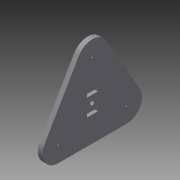
# Autodesk Inventor part: RibEnd
Saved by Autodesk Inventor 2015 (Build 190159000, 159)
## iProperties
Created: 2014-11-09
Part Number: RibEnd
Material: Generic
Document SubType Name: Modeling
Designer: Ryan
Density: 1 g/cm^3
Appearance: Default
Author: Ryan
Autodesk Inventor part; units mm, degrees
ref_plane "YZ Plane" through (0, 0, 0) normal (1, 0, 0) x (0, 1, 0)
ref_plane "XZ Plane" through (0, 0, 0) normal (0, 1, 0) x (-1, 0, 0)
ref_plane "XY Plane" through (0, 0, 0) normal (0, 0, 1) x (1, 0, 0)
sketch "Sketch1" plane through (0, 0, 0) normal (1, 0, 0) x (0, 1, 0)
  line L0 (2.9851, 0) -> (0, 0) construction
  line L1 (0, 0) -> (0, 4.2) construction
  circle A0 centre (0, 0) radius 1.425
  circle A1 centre (25.125, 0) radius 10
  circle A2 centre (-12.5625, 21.7589) radius 10
  circle A3 centre (-12.5625, -21.7589) radius 10
  line L2 (-7.5625, 30.4191) -> (30.125, 8.6603)
  line L3 (-22.5625, 21.7589) -> (-22.5625, -21.7589)
  line L4 (30.125, -8.6603) -> (-7.5625, -30.4191)
  line L5 (0, 0) -> (-12.5625, 21.7589) construction
  line L6 (-12.5625, 21.7589) -> (-12.5625, -21.7589) construction
  line L7 (-12.5625, 21.7589) -> (25.125, 0) construction
  line L8 (6.5, 3.5) -> (4.5, 3.5)
  line L9 (4.5, 3.5) -> (4.5, -3.5)
  line L10 (4.5, -3.5) -> (6.5, -3.5)
  line L11 (6.5, -3.5) -> (6.5, 3.5)
  line L12 (-4.5, 3.5) -> (-6.5, 3.5)
  line L13 (-6.5, 3.5) -> (-6.5, -3.5)
  line L14 (-6.5, -3.5) -> (-4.5, -3.5)
  line L15 (-4.5, -3.5) -> (-4.5, 3.5)
  dimension "d0" = 25.125
  dimension "d1" = 25.125
  dimension "d2" = 60
  dimension "d3" = 20
  dimension "d4" = 20
  dimension "d5" = 2.85
  dimension "d6" = 2
  dimension "d7" = 7
  dimension "d8" = 4.5
  constraints: 32 end point, 6 point on circle, 6 tangent, 4 centre point, 4 parallel, 3 horizontal, 2 perpendicular, 2 vertical, 1 coincident, 1 point on line, 1 symmetric about line, 6 other
  measures "d0" distance of L7.end L0.end
  measures "d1" distance of L5.start L5.end
  measures "d2" angle of L6 L7
  measures "d3" diameter of A1
  measures "d4" diameter of A3
  measures "d5" diameter of A0
  measures "d6" distance of L9.end L10.end
  measures "d7" distance of L10.end L8.start
  measures "d8" distance from line of L9 L0.end
extrude "Extrusion1" add sketch "Sketch1" against normal blind 3
sketch "Sketch6" plane through (0, 0, 0) normal (1, 0, 0) x (0, 0, -1)
  circle A0 centre (0, 25.125) radius 0.5
  circle A1 centre (-21.7589, -12.5625) radius 0.5
  circle A2 centre (21.7589, -12.5625) radius 0.5
  line L0 (0, 0) -> (0, 25.125)
  line L1 (0, 25.125) -> (-21.7589, -12.5625)
  line L2 (-21.7589, -12.5625) -> (21.7589, -12.5625)
  line L3 (21.7589, -12.5625) -> (0, 0)
  dimension "d32" = 25.125
  dimension "d33" = 25.125
  dimension "d34" = 60
  dimension "d35" = 1
  dimension "d36" = 1
  dimension "d37" = 1
  constraints: 8 end point, 3 centre point, 1 horizontal, 1 symmetric about line, 1 vertical
  measures "d32" distance of L2.end L0.start
  measures "d33" distance of L0.start L0.end
  measures "d34" angle of L2 L1
  measures "d35" diameter of A1
  measures "d36" diameter of A0
  measures "d37" diameter of A2
hole "Hole1" at (0, 25.125, 0) at (0, -12.5625, 21.7589) at (0, -12.5625, -21.7589) direction (-1, 0, 0) diameter 1 end through all
body "Solid1"
